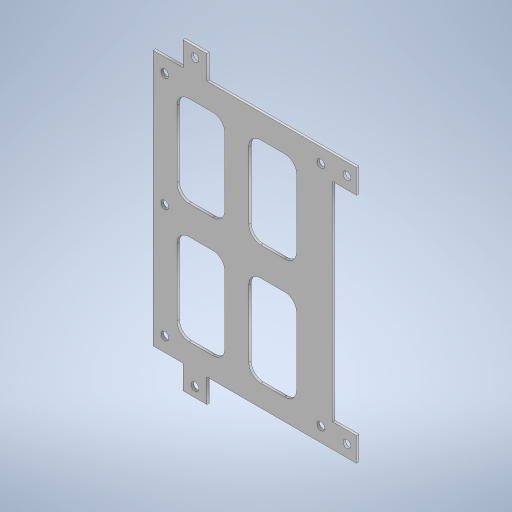
# Autodesk Inventor part: left
Saved by Autodesk Inventor 2023 (Build 270158000, 158)
## iProperties
Created: 2023-05-25
Part Number: left
Material: 一般
Document SubType Name: Sheet Metal
Designer: 310611102
Density: 1 g/cm^3
Sheet Metal Rule: Default_mm
Appearance: 預設
Author: 310611102
Autodesk Inventor part; units mm, degrees
ref_plane "YZ Plane" through (0, 0, 0) normal (1, 0, 0) x (0, 1, 0)
ref_plane "XZ Plane" through (0, 0, 0) normal (0, 1, 0) x (-1, 0, 0)
ref_plane "XY Plane" through (0, 0, 0) normal (0, 0, 1) x (1, 0, 0)
sketch "Sketch2" plane through (0, 0, 0) normal (0, 0, 1) x (1, 0, 0)
  line L0 (-37.5, 53.5) -> (37.5, 53.5)
  line L1 (37.5, 53.5) -> (37.5, -53.5)
  line L2 (37.5, -53.5) -> (-37.5, -53.5)
  line L3 (-37.5, -53.5) -> (-37.5, 53.5)
  line L4 (-37.5, 53.5) -> (37.5, -53.5) construction
  line L5 (37.5, 53.5) -> (-37.5, -53.5) construction
  line L6 (-22.5, 43.5) -> (-12.5, 43.5)
  line L7 (-7.5, 38.5) -> (-7.5, 10.5)
  line L8 (-12.5, 5.5) -> (-22.5, 5.5)
  line L9 (-27.5, 10.5) -> (-27.5, 38.5)
  line L10 (-27.5, 43.5) -> (-7.5, 5.5) construction
  line L11 (-7.5, 43.5) -> (-27.5, 5.5) construction
  arc A0 (-22.5, 43.5) -> (-27.5, 38.5) centre (-22.5, 38.5) ccw
  arc A1 (-7.5, 38.5) -> (-12.5, 43.5) centre (-12.5, 38.5) ccw
  arc A2 (-12.5, 5.5) -> (-7.5, 10.5) centre (-12.5, 10.5) ccw
  arc A3 (-27.5, 10.5) -> (-22.5, 5.5) centre (-22.5, 10.5) ccw
  line L12 (7.5, 43.5) -> (17.5, 43.5)
  arc A4 (22.5, 38.5) -> (17.5, 43.5) centre (17.5, 38.5) ccw
  arc A5 (17.5, 5.5) -> (22.5, 10.5) centre (17.5, 10.5) ccw
  arc A6 (2.5, 10.5) -> (7.5, 5.5) centre (7.5, 10.5) ccw
  arc A7 (7.5, 43.5) -> (2.5, 38.5) centre (7.5, 38.5) ccw
  line L13 (22.5, 38.5) -> (22.5, 10.5)
  line L14 (17.5, 5.5) -> (7.5, 5.5)
  line L15 (2.5, 10.5) -> (2.5, 38.5)
  line L16 (22.5, 43.5) -> (2.5, 5.5) construction
  line L17 (2.5, 43.5) -> (22.5, 5.5) construction
  line L18 (-22.5, -6.5) -> (-12.5, -6.5)
  arc A8 (-7.5, -11.5) -> (-12.5, -6.5) centre (-12.5, -11.5) ccw
  arc A9 (-12.5, -44.5) -> (-7.5, -39.5) centre (-12.5, -39.5) ccw
  arc A10 (-27.5, -39.5) -> (-22.5, -44.5) centre (-22.5, -39.5) ccw
  arc A11 (-22.5, -6.5) -> (-27.5, -11.5) centre (-22.5, -11.5) ccw
  line L19 (-7.5, -11.5) -> (-7.5, -39.5)
  line L20 (-12.5, -44.5) -> (-22.5, -44.5)
  line L21 (-27.5, -39.5) -> (-27.5, -11.5)
  line L22 (-7.5, -6.5) -> (-27.5, -44.5) construction
  line L23 (-27.5, -6.5) -> (-7.5, -44.5) construction
  line L24 (7.5, -6.5) -> (17.5, -6.5)
  arc A12 (22.5, -11.5) -> (17.5, -6.5) centre (17.5, -11.5) ccw
  arc A13 (17.5, -44.5) -> (22.5, -39.5) centre (17.5, -39.5) ccw
  arc A14 (2.5, -39.5) -> (7.5, -44.5) centre (7.5, -39.5) ccw
  arc A15 (7.5, -6.5) -> (2.5, -11.5) centre (7.5, -11.5) ccw
  line L25 (22.5, -11.5) -> (22.5, -39.5)
  line L26 (17.5, -44.5) -> (7.5, -44.5)
  line L27 (2.5, -39.5) -> (2.5, -11.5)
  line L28 (22.5, -6.5) -> (2.5, -44.5) construction
  line L29 (2.5, -6.5) -> (22.5, -44.5) construction
  circle A16 centre (-32.6, 0) radius 1.6
  line L30 (0, 0) -> (0, 8.2468)
  circle A17 centre (-32.6, -47.5) radius 1.6
  line L31 (0, 0) -> (-8.4645, 0)
  circle A18 centre (32.6, -47.5) radius 1.6
  circle A19 centre (-32.6, 47.5) radius 1.6
  circle A20 centre (32.6, 47.5) radius 1.6
  point P0 (-17.5, 24.5)
  point P1 (12.5, 24.5)
  point P2 (-17.5, -25.5)
  point P3 (12.5, -25.5)
  dimension "d27" = 107
  dimension "d28" = 75
  dimension "d29" = 20
  dimension "d30" = 38
  dimension "d31" = 5
  dimension "d34" = 30
  dimension "d37" = 50
  dimension "d40" = 10
  dimension "d41" = 10
  dimension "d42" = 3.2
  dimension "d43" = 4.9
  dimension "d44" = 3.2
  dimension "d45" = 4.9
  dimension "d46" = 6
  measures "d27" distance of L0.end L1.end
  measures "d28" distance of L0.start L0.end
  measures "d29" distance of L10.start L11.start
  measures "d30" distance of L11.end L10.start
  measures "d31" radius of A0
  measures "d34" distance of L6.start L12.start
  measures "d37" distance of L6.start L18.start
  measures "d40" distance between parallel lines of L0 L6
  measures "d41" distance between parallel lines of L3 L9
  measures "d42" diameter of A16
  measures "d43" distance from line of L3 A16.centre
  measures "d44" diameter of A17
  measures "d45" distance from line of L3 A17.centre
  measures "d46" distance from line of L2 A17.centre
sketch "Sketch3" plane through (0, 0, 1) normal (0, 0, 1) x (1, 0, 0)
  arc A0 (22.5, -11.5) -> (17.5, -6.5) centre (17.5, -11.5) ccw
  line L0 (22.5, -11.5) -> (22.5, -39.5)
  arc A1 (17.5, -44.5) -> (22.5, -39.5) centre (17.5, -39.5) ccw
  line L1 (17.5, -44.5) -> (7.5, -44.5)
  arc A2 (2.5, -39.5) -> (7.5, -44.5) centre (7.5, -39.5) ccw
  line L2 (2.5, -39.5) -> (2.5, -11.5)
  arc A3 (7.5, -6.5) -> (2.5, -11.5) centre (7.5, -11.5) ccw
  line L3 (7.5, -6.5) -> (17.5, -6.5)
  arc A4 (-7.5, -11.5) -> (-12.5, -6.5) centre (-12.5, -11.5) ccw
  line L4 (-7.5, -11.5) -> (-7.5, -39.5)
  arc A5 (-12.5, -44.5) -> (-7.5, -39.5) centre (-12.5, -39.5) ccw
  line L5 (-12.5, -44.5) -> (-22.5, -44.5)
  arc A6 (-27.5, -39.5) -> (-22.5, -44.5) centre (-22.5, -39.5) ccw
  line L6 (-27.5, -39.5) -> (-27.5, -11.5)
  arc A7 (-22.5, -6.5) -> (-27.5, -11.5) centre (-22.5, -11.5) ccw
  line L7 (-22.5, -6.5) -> (-12.5, -6.5)
  arc A8 (22.5, 38.5) -> (17.5, 43.5) centre (17.5, 38.5) ccw
  line L8 (22.5, 38.5) -> (22.5, 10.5)
  arc A9 (17.5, 5.5) -> (22.5, 10.5) centre (17.5, 10.5) ccw
  line L9 (17.5, 5.5) -> (7.5, 5.5)
  arc A10 (2.5, 10.5) -> (7.5, 5.5) centre (7.5, 10.5) ccw
  line L10 (2.5, 10.5) -> (2.5, 38.5)
  arc A11 (7.5, 43.5) -> (2.5, 38.5) centre (7.5, 38.5) ccw
  line L11 (7.5, 43.5) -> (17.5, 43.5)
  arc A12 (-22.5, 43.5) -> (-27.5, 38.5) centre (-22.5, 38.5) ccw
  line L12 (-22.5, 43.5) -> (-12.5, 43.5)
  arc A13 (-7.5, 38.5) -> (-12.5, 43.5) centre (-12.5, 38.5) ccw
  line L13 (-7.5, 38.5) -> (-7.5, 10.5)
  arc A14 (-12.5, 5.5) -> (-7.5, 10.5) centre (-12.5, 10.5) ccw
  line L14 (-12.5, 5.5) -> (-22.5, 5.5)
  arc A15 (-27.5, 10.5) -> (-22.5, 5.5) centre (-22.5, 10.5) ccw
  line L15 (-27.5, 10.5) -> (-27.5, 38.5)
  circle A16 centre (32.6, 47.5) radius 1.6
  circle A17 centre (-32.6, 47.5) radius 1.6
  circle A18 centre (32.6, -47.5) radius 1.6
  circle A19 centre (-32.6, -47.5) radius 1.6
  circle A20 centre (-32.6, 0) radius 1.6
  line L16 (37.5, 53.5) -> (37.5, -53.5)
  line L17 (-37.5, 53.5) -> (37.5, 53.5)
  line L18 (-37.5, -53.5) -> (-37.5, 53.5)
  line L19 (37.5, -53.5) -> (-37.5, -53.5)
  line L20 (-37.5, 53.5) -> (37.5, 53.5)
  line L21 (-25, 63.5) -> (-15, 63.5)
  line L22 (-15, 63.5) -> (-15, 53.5)
  line L23 (-15, 53.5) -> (-25, 53.5)
  line L24 (-25, 53.5) -> (-25, 63.5)
  line L25 (37.5, 53.5) -> (47.5, 53.5)
  line L26 (47.5, 53.5) -> (47.5, 43.5)
  line L27 (47.5, 43.5) -> (37.5, 43.5)
  line L28 (0, 0) -> (8, 0)
  circle A21 centre (-20, 59.5) radius 1.6
  circle A22 centre (43.5, 48.5) radius 1.6
  line L29 (-25, -63.5) -> (-15, -63.5)
  line L30 (-15, -63.5) -> (-15, -53.5)
  line L31 (-15, -53.5) -> (-25, -53.5)
  line L32 (-25, -53.5) -> (-25, -63.5)
  line L33 (37.5, -53.5) -> (47.5, -53.5)
  line L34 (47.5, -53.5) -> (47.5, -43.5)
  line L35 (47.5, -43.5) -> (37.5, -43.5)
  circle A23 centre (-20, -59.5) radius 1.6
  circle A24 centre (43.5, -48.5) radius 1.6
  line L36 (37.5, 53.5) -> (37.5, 43.5)
  line L37 (37.5, 53.5) -> (37.5, -53.5)
  line L38 (37.5, -53.5) -> (37.5, -43.5)
  point P0 (-20, 63.5)
  point P1 (47.5, 48.5)
  point P2 (-20, -63.5)
  point P3 (47.5, -48.5)
  point P4 (0, 53.5)
  point P5 (0, 53.5)
  dimension "d65" = 4
  dimension "d66" = 10
  dimension "d67" = 10
  dimension "d68" = 10
  dimension "d69" = 10
  dimension "d70" = 4
  dimension "d71" = 3.2
  dimension "d72" = 3.2
  dimension "d77" = 5
  dimension "d78" = 97
  dimension "d79" = 43.5
  dimension "d81" = 119
  dimension "d83" = 20
  measures "d65" distance from line of L26 A22.centre
  measures "d66" distance of L25.end L26.end
  measures "d67" distance between parallel lines of L16 L26
  measures "d68" distance of L21.start L21.end
  measures "d69" distance of L21.end L22.end
  measures "d70" distance from line of L21 A21.centre
  measures "d71" diameter of A21
  measures "d72" diameter of A22
  measures "d77" distance from line of L17 A22.centre
  measures "d78" diameter of A22.centre L28
  measures "d79" horizontal distance of A22.centre L28.start
  measures "d81" distance of A23.centre A21.centre
  measures "d83" horizontal distance of A21.centre point (0, 53.5)
extrude "Plate2" add sketch "Sketch2" along normal blind 1
sheet face with bend "Face3" sketch "Sketch3" thickness 1 toward (0, 0, -1) bend radius 1 relief straight relief width 1 relief depth 0.5 contours L25 L26 L27 L16 | L17 L24 L21 L22 | L35 L34 L33 L16 | L30 L29 L32 L19
bend "Bend1"
equation "\"d14\" = 厚度"
equation "\"d53\" = 折彎半徑"
equation "\"d54\" = 折彎離隙寬度"
equation "\"d56\" = 最小剩餘"
equation "\"d55\" = 折彎離隙深度"
equation "\"d57\" = 轉移半徑"
equation "\"折彎半徑\" = 厚度"
equation "\"折彎離隙寬度\" = 厚度"
equation "\"折彎離隙深度\" = 0.5 * 厚度"
equation "\"轉角離隙大小\" = 4 * 厚度"
equation "\"最小剩餘\" = 2 * 厚度"
equation "\"轉移半徑\" = 折彎半徑"
equation "\"Jacobi半徑大小\" = 折彎半徑"
equation "\"間隙大小\" = 厚度"
equation "\"厚度\" = 1"
body "Solid1"
